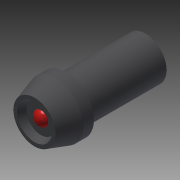
# Autodesk Inventor part: LED_Inset
Saved by Autodesk Inventor 2014 (Build 180170000, 170)
## iProperties
Created: 2015-01-07
Part Number: LED_Inset
Material: Generic
Document SubType Name: Modeling
Designer: Owner
Density: 1 g/cm^3
Appearance: Gray
Author: Owner
Autodesk Inventor part; units mm, degrees
ref_plane "YZ Plane" through (0, 0, 0) normal (1, 0, 0) x (0, 1, 0)
ref_plane "XZ Plane" through (0, 0, 0) normal (0, 1, 0) x (-1, 0, 0)
ref_plane "XY Plane" through (0, 0, 0) normal (0, 0, 1) x (1, 0, 0)
sketch "Sketch1" plane through (0, 0, 0) normal (0, 0, 1) x (1, 0, 0)
  circle A0 centre (0, 0) radius 4
  dimension "d0" = 8
  constraints: 1 centre point, 1 coincident
  measures "d0" diameter of A0
extrude "Extrusion1" add sketch "Sketch1" along normal blind 21
sketch "Sketch2" plane through (0, 0, 21) normal (0, 0, 1) x (1, 0, 0)
  circle A0 centre (0, 0) radius 4 projected
  circle A1 centre (0, 0) radius 5.25
  dimension "d3" = 10.5
  constraints: 1 centre point, 1 coincident
  measures "d3" diameter of A1
extrude "Extrusion2" add sketch "Sketch2" against normal blind 6 contours A0 | A1
chamfer "Chamfer1" distance 4 distance2 1.25 1 edges at (-5.25, 0, 21) measured on face at (5.182, -0.8422, 17)
sketch "Sketch3" plane through (0, 0, 0) normal (1, 0, 0) x (0, 1, 0)
  arc A0 (1.3613, 19.7935) -> (0, 20.6635) centre (0, 19.1635) ccw
  line L0 (1.3613, 19.7935) -> (2.7354, 19.7935)
  line L1 (2.7354, 19.7935) -> (3.3091, 20.9972)
  line L2 (3.3091, 20.9972) -> (3.3091, 22.2347)
  line L3 (3.3091, 22.2347) -> (0, 22.2347)
  line L4 (0, 22.2347) -> (0, 20.6635)
  point P0 (0, 0)
  dimension "d9" = 3
  dimension "d10" = 2.8704
  constraints: 10 end point, 2 parallel, 2 point on circle, 1 centre point, 1 horizontal, 1 perpendicular
  measures "d9" diameter of A0
  measures "d10" distance of L4.end L0.end
revolve "Revolution1" cut sketch "Sketch3" angle 360 about axis through (0, 0, 22.2347) along (0, 0, -1)
body "Solid1"
